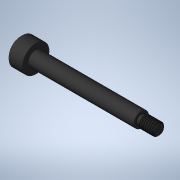
# Autodesk Inventor part: SCLBRU5-35.0_D
Saved by Autodesk Inventor 2021 (Build 250183000, 183)
## iProperties
Created: 2025-08-07
Part Number: SCLBRU5-35.0_D
Material: Generic
Catalog Web Link: www.cadenas.de
Description: CLBR, CLBRH, PCLBR, PCLBRH, GCLBR, SCLBR, SCLBRH, GSCLBR, CLBRU, CLBRHU, PCLBRU, PCLBRHU, GCLBRU, SCLBRU, SCLBRHU, GSCLBRU_D-Hinge Pins - Lock Nut Type with Hexagon Socket Head
Vendor: MISUMI
Document SubType Name: Modeling
Designer: psAdmin
Manufacturer: MISUMI
Mass: 1.05743 g
Surface Area: 9.05155 cm^2
Volume: 1.05743 cm^3
Density: 1 g/cm^3
Appearance: PSOLRGB-175-175-175
Category: PARTsolutions
Company: MISUMI
Title: SCLBRU5-35.0
Author: Cadenas PARTsolutions
Comments: Hinge Pins - Lock Nut Type with Hexagon Socket Head
PSOL_IDENT_0: {$CADENAS_DATA/23d-libs/misumi/metric/13_cantilever_shafts/clbr/clbr_d.prj},333 {VTYP=3D},{NB=SCLBRU
PSOL_IDENT_1: 5-35.0_D},{LINA=SCLBRU5-35.0},{NN=CLBR, CLBRH, PCLBR, PCLBRH, GCLBR, SCLBR, SCLBRH, GSCLBR, CLBRU, C
PSOL_IDENT_2: LBRHU, PCLBRU, PCLBRHU, GCLBRU, SCLBRU, SCLBRHU, GSCLBRU_D},{DATE=21.04.2022 08:37:10},{GEOMDATE=16.
PSOL_IDENT_3: 06.2021 04:18:25},{VERSION=},{LINEID=30},{WBVAR=MAT,HARD,ST,AC,L,ALT3,ALT2,MC,ALT1,FC,ALT4},{WBNUMER
PSOL_IDENT_4: IC=L,MC,FC}  {NB=SCLBRU5-35.0_D},{LINA=SCLBRU5-35.0},{KT=DUMMY},{PN=SCLBRU5-35.0},{TYPE=SCLBRU},{MAT=
PSOL_IDENT_5: SUS304},{HARD=1},{HARDALG= '1', '-' },{ST=},{STALG= '', '-' },{AC=UN},{ACALG= 'SN', 'Standard Nuts',
PSOL_IDENT_6: 'UN', 'U-Nuts' },{MATAC1=304 Stainless Steel (UNUTS)},{MATAC2=0},{STAC=0},{D=5},{L=35.0},{L1=[10.0:
PSOL_IDENT_7: 100.0/0.1]},{LPN=35.0},{LPN1=35},{LPN2=0},{ALT3=},{A=9},{T=5},{ALT2=},{ALT2ALG= '' , 'Not applicable'
PSOL_IDENT_8: },{ALT2PN=},{MC=0},{MCALG=0},{M=M4},{M1=4},{M3D=4},{ALT1=},{ALT1ALG= '', 'w/o FC (Thread Part Lengt
PSOL_IDENT_9: h)', '-FC', 'with FC (Thread Part Length)' },{ALT1PN=},{FC=0},{FCALG=0},{FCMIN1=4},{FCMAX1=5},{FCMIN
PSOL_IDENT_10: 2=7.000},{FCMAX2=12},{F=6},{F3D=6},{B=2.5},{E=2},{UU=4.9},{NN=1.5},{NUT=M3x0.7},{ALT4=},{HC=3.50},{G
PSOL_IDENT_11: G=1.2},{RR=0.3},{FF=3.1},{MAC=4},{BAC=7},{TAC=3.2},{CS=One side}
NB: SCLBRU5-35.0_D
NN: 1.5
NT: Hinge Pins - Lock Nut Type with Hexagon Socket Head
NBSYN: $PN._D
LINA: SCLBRU5-35.0
CATALOG: Misumi
PN: SCLBRU5-35.0
MAT: SUS304
HARD: -
ST: -
AC: U-Nuts
D: 5
L: 35
ALT3: w/o LKC (L Dimension Tolerance)
A: 9
T: 5
ALT2: Not applicable
MC: 0
M: M4
ALT1: w/o FC (Thread Part Length)
FC: 0
F: 6
B: 2.5
E: 2
UU: 4.9
NUT: M3x0.7
ALT4: w/o HC (Shoulder Diameter Cut)
SUPPLIER: MISUMI
ARTICLENO: SCLBRU5-35.0_D
BOMINFO: SCLBRU5-35.0
CREATOR: CADENAS GmbH
Autodesk Inventor part; units mm, degrees
sketch "Sketch_1" plane through (0, 0, 0) normal (0, 0, 1) x (1, 0, 0)
  line L0 (41, 0) -> (-5, 0)
  line L1 (-2.2783, 0) -> (-3, 1.25)
  line L2 (-3, 1.25) -> (-5, 1.25)
  line L3 (-5, 1.25) -> (-5, 4)
  line L4 (-5, 4) -> (-4.5, 4.5)
  line L5 (-4.5, 4.5) -> (0, 4.5)
  line L6 (0, 4.5) -> (0, 2.45)
  line L7 (0, 2.45) -> (1.5, 2.45)
  line L8 (1.5, 2.45) -> (1.5, 2.5)
  line L9 (1.5, 2.5) -> (35, 2.5)
  line L10 (35, 2.5) -> (35, 1.85)
  arc A0 (35, 1.85) -> (35.3, 1.55) centre (35.3, 1.85) ccw
  line L11 (35.3, 1.55) -> (35.9, 1.55)
  arc A1 (35.9, 1.55) -> (36.2, 1.85) centre (35.9, 1.85) ccw
  line L12 (36.2, 1.85) -> (36.2, 2)
  line L13 (36.2, 2) -> (40.5705, 2)
  line L14 (40.5705, 2) -> (41, 1.5705)
  line L15 (41, 1.5705) -> (41, 0)
  line L16 (41, 0) -> (-2.2783, 0)
  constraints: 34 end point, 4 point on circle, 2 centre point
revolve "Revolution1" add sketch "Sketch_1" angle 360 about axis through (41, 0, 0) along (1, 0, 0)
thread "Thread1" size "M4x0.7" class "6g" standard "ISO Metric profile" full length
sketch "Sketch_2" plane through (-5, 0, 0) normal (1, 0, 0) x (0, 0, -1)
  line L0 (-1.25, -0.7217) -> (0, -1.4434)
  line L1 (0, -1.4434) -> (1.25, -0.7217)
  line L2 (1.25, -0.7217) -> (1.25, 0.7217)
  line L3 (1.25, 0.7217) -> (0, 1.4434)
  line L4 (0, 1.4434) -> (-1.25, 0.7217)
  line L5 (-1.25, 0.7217) -> (-1.25, -0.7217)
  constraints: 12 end point
extrude "Extrusion1" cut sketch "Sketch_2" along normal blind 2
ref_plane "pin_to_nut_XY" through (36.7, 0, 0) normal (1, 0, 0) x (0, 0, -1)
ref_plane "pin_to_nut_YZ" through (36.7, 0, 0) normal (0, 0, -1) x (0, 1, 0)
ref_plane "pin_to_nut_ZX" through (36.7, 0, 0) normal (0, 1, 0) x (1, 0, 0)
body "Solid1"
